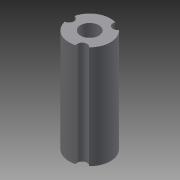
# Autodesk Inventor part: slip_ring_internal
Saved by Autodesk Inventor 2015 (Build 190159000, 159)
## iProperties
Created: 2017-12-05
Part Number: slip_ring_internal
Material: Generic
Document SubType Name: Modeling
Designer: Anshul
Density: 1 g/cm^3
Appearance: Default
Author: Anshul
Autodesk Inventor part; units mm, degrees
ref_plane "YZ Plane" through (0, 0, 0) normal (1, 0, 0) x (0, 1, 0)
ref_plane "XZ Plane" through (0, 0, 0) normal (0, 1, 0) x (-1, 0, 0)
ref_plane "XY Plane" through (0, 0, 0) normal (0, 0, 1) x (1, 0, 0)
sketch "Sketch1" plane through (0, 0, 0) normal (0, 1, 0) x (-1, 0, 0)
  circle A0 centre (7.25, 0) radius 1.75
  circle A1 centre (-3.625, 6.2787) radius 1.75
  circle A2 centre (-3.625, -6.2787) radius 1.75
  circle A3 centre (0, 0) radius 3.2
  arc A4 (-2.0149, -6.9644) -> (7.0388, -1.7372) centre (0, 0) ccw
  arc A5 (7.0388, 1.7372) -> (-2.0149, 6.9644) centre (0, 0) ccw
  arc A6 (-5.0239, 5.2272) -> (-5.0239, -5.2272) centre (0, 0) ccw
  dimension "d24" = 3.5
  dimension "d25" = 3.5
  dimension "d26" = 3.5
  dimension "d27" = 6.4
  constraints: 12 point on circle, 7 centre point, 1 coincident
  measures "d24" diameter of A0
  measures "d25" diameter of A1
  measures "d26" diameter of A2
  measures "d27" diameter of A3
extrude "Extrusion3" add sketch "Sketch1" along normal blind 36 contours A0 A4 A2 A6 A1 A5
body "Solid3"
